Autodesk Fusion 360 part; units mm, degrees
note: some values were not read from the file. Chosen so that the rebuilt part matches the saved one: which bodies a step acts on.
(part 3 of 3)
  line L1048 (193.125, 122.3141) -> (193.125, 116.0647)
  line L1049 (193.125, 116.0647) -> (191.8255, 116.0647)
  line L1050 (191.8255, 116.0647) -> (191.8255, 120.6243)
  line L1051 (191.8255, 120.6243) -> (189.2661, 120.6243)
  line L1052 (189.2661, 120.6243) -> (189.2661, 116.8805)
  line L1053 (189.2661, 116.8805) -> (187.9666, 116.8805)
  line L1054 (187.9666, 116.8805) -> (187.9666, 120.6243)
  line L1055 (187.9666, 120.6243) -> (185.752, 120.6243)
  line L1056 (185.752, 120.6243) -> (185.752, 116.2104)
  line L1057 (185.752, 116.2104) -> (184.4524, 116.2104)
  line L1058 (184.4524, 116.2104) -> (184.4524, 122.3141)
  line L1059 (184.4524, 122.3141) -> (193.125, 122.3141)
  spline S282 degree 3 poles (193.2842, 101.9604) (193.2842, 99.8627) (192.1835, 98.6537) (189.8098, 98.6537) knots 0 0 0 0 1 1 1 1
  line L1060 (189.8098, 98.6537) -> (184.4525, 98.6537)
  line L1061 (184.4525, 98.6537) -> (184.4525, 100.2706)
  line L1062 (184.4525, 100.2706) -> (189.9292, 100.2706)
  spline S283 degree 3 poles (189.9292, 100.2706) (191.3481, 100.2706) (191.9448, 100.9261) (191.9448, 101.9604) knots 0 0 0 0 1 1 1 1
  spline S284 degree 3 poles (191.9448, 101.9604) (191.9448, 102.9801) (191.3481, 103.6065) (189.9292, 103.6065) knots 0 0 0 0 1 1 1 1
  line L1063 (189.9292, 103.6065) -> (184.4525, 103.6065)
  line L1064 (184.4525, 103.6065) -> (184.4525, 105.2963)
  line L1065 (184.4525, 105.2963) -> (189.8098, 105.2963)
  spline S285 degree 3 poles (189.8098, 105.2963) (192.1835, 105.2963) (193.2842, 104.0435) (193.2842, 101.9604) knots 0 0 0 0 1 1 1 1
  line L1066 (193.125, 87.7978) -> (193.125, 86.1809)
  line L1067 (193.125, 86.1809) -> (189.3324, 86.1809)
  spline S286 degree 3 poles (189.3324, 86.1809) (188.3644, 86.1809) (187.3301, 86.3411) (186.4018, 86.414) knots 0 0 0 0 1 1 1 1
  line L1068 (186.4018, 86.414) -> (186.4018, 86.3703)
  line L1069 (186.4018, 86.3703) -> (188.2451, 85.5108)
  line L1070 (188.2451, 85.5108) -> (193.125, 82.9906)
  line L1071 (193.125, 82.9906) -> (193.125, 81.2134)
  line L1072 (193.125, 81.2134) -> (184.4525, 81.2134)
  line L1073 (184.4525, 81.2134) -> (184.4525, 82.8304)
  line L1074 (184.4525, 82.8304) -> (188.2185, 82.8304)
  spline S287 degree 3 poles (188.2185, 82.8304) (189.1866, 82.8304) (190.2872, 82.6702) (191.1757, 82.5973) knots 0 0 0 0 1 1 1 1
  line L1075 (191.1757, 82.5973) -> (191.1757, 82.641)
  line L1076 (191.1757, 82.641) -> (189.3192, 83.5005)
  line L1077 (189.3192, 83.5005) -> (184.4525, 86.0207)
  line L1078 (184.4525, 86.0207) -> (184.4525, 87.7979)
  line L1079 (184.4525, 87.7979) -> (193.125, 87.7978)
  line L1080 (193.125, 70.212) -> (193.125, 68.493)
  line L1081 (193.125, 68.493) -> (190.5657, 68.493)
  line L1082 (190.5657, 68.493) -> (189.0009, 67.1383)
  line L1083 (189.0009, 67.1383) -> (193.125, 64.7347)
  line L1084 (193.125, 64.7347) -> (193.125, 62.8555)
  line L1085 (193.125, 62.8555) -> (187.8207, 66.104)
  line L1086 (187.8207, 66.104) -> (184.4525, 63.1614)
  line L1087 (184.4525, 63.1614) -> (184.4525, 65.0552)
  line L1088 (184.4525, 65.0552) -> (188.3909, 68.4494)
  line L1089 (188.3909, 68.4494) -> (188.3909, 68.4931)
  line L1090 (188.3909, 68.4931) -> (184.4525, 68.4931)
  line L1091 (184.4525, 68.4931) -> (184.4525, 70.212)
  line L1092 (184.4525, 70.212) -> (193.125, 70.212)
  spline S288 degree 3 poles (193.2842, 49.5524) (193.2842, 47.4547) (192.1835, 46.2456) (189.8098, 46.2456) knots 0 0 0 0 1 1 1 1
  line L1093 (189.8098, 46.2456) -> (184.4525, 46.2456)
  line L1094 (184.4525, 46.2456) -> (184.4525, 47.8626)
  line L1095 (184.4525, 47.8626) -> (189.9292, 47.8626)
  spline S289 degree 3 poles (189.9292, 47.8626) (191.3481, 47.8626) (191.9448, 48.5181) (191.9448, 49.5524) knots 0 0 0 0 1 1 1 1
  spline S290 degree 3 poles (191.9448, 49.5524) (191.9448, 50.5721) (191.3481, 51.1985) (189.9292, 51.1985) knots 0 0 0 0 1 1 1 1
  line L1096 (189.9292, 51.1985) -> (184.4525, 51.1985)
  line L1097 (184.4525, 51.1985) -> (184.4525, 52.8883)
  line L1098 (184.4525, 52.8883) -> (189.8098, 52.8883)
  spline S291 degree 3 poles (189.8098, 52.8883) (192.1835, 52.8883) (193.2842, 51.6355) (193.2842, 49.5524) knots 0 0 0 0 1 1 1 1
  line L1099 (193.125, 35.419) -> (193.125, 33.7292)
  line L1100 (193.125, 33.7292) -> (189.2794, 33.7292)
  line L1101 (189.2794, 33.7292) -> (189.2794, 30.4661)
  line L1102 (189.2794, 30.4661) -> (193.125, 30.4661)
  line L1103 (193.125, 30.4661) -> (193.125, 28.7763)
  line L1104 (193.125, 28.7763) -> (184.4525, 28.7763)
  line L1105 (184.4525, 28.7763) -> (184.4525, 30.4661)
  line L1106 (184.4525, 30.4661) -> (187.9401, 30.4661)
  line L1107 (187.9401, 30.4661) -> (187.9401, 33.7292)
  line L1108 (187.9401, 33.7292) -> (184.4525, 33.7292)
  line L1109 (184.4525, 33.7292) -> (184.4525, 35.419)
  line L1110 (184.4525, 35.419) -> (193.125, 35.419)
  line L1111 (193.125, 17.7748) -> (193.125, 16.085)
  line L1112 (193.125, 16.085) -> (189.7303, 16.085)
  line L1113 (189.7303, 16.085) -> (189.7303, 14.6574)
  line L1114 (189.7303, 14.6574) -> (193.125, 12.618)
  line L1115 (193.125, 12.618) -> (193.125, 10.7096)
  line L1116 (193.125, 10.7096) -> (189.5048, 12.9822)
  spline S292 degree 3 poles (189.5048, 12.9822) (189.1468, 11.8459) (188.3379, 11.0884) (187.0251, 11.0884) knots 0 0 0 0 1 1 1 1
  spline S293 degree 3 poles (187.0251, 11.0884) (185.089, 11.0884) (184.4525, 12.618) (184.4525, 14.5991) knots 0 0 0 0 1 1 1 1
  line L1117 (184.4525, 14.5991) -> (184.4525, 17.7748)
  line L1118 (184.4525, 17.7748) -> (193.125, 17.7748)
  line L1119 (188.5103, 16.085) -> (185.6857, 16.085)
  line L1120 (185.6857, 16.085) -> (185.6857, 14.7739)
  spline S294 degree 3 poles (185.6857, 14.7739) (185.6857, 13.4629) (186.0305, 12.7491) (187.0251, 12.7491) knots 0 0 0 0 1 1 1 1
  spline S295 degree 3 poles (187.0251, 12.7491) (188.0063, 12.7491) (188.5103, 13.4628) (188.5103, 14.7739) knots 0 0 0 0 1 1 1 1
  line L1121 (188.5103, 14.7739) -> (188.5103, 16.085)
  line L1122 (17.9457, 85.157) -> (17.9457, 83.9457)
  line L1123 (17.9457, 83.9457) -> (19.921, 83.9457)
  line L1124 (19.921, 83.9457) -> (19.921, 85.157)
  line L1125 (19.921, 85.157) -> (17.9457, 85.157)
  line L1126 (36.9623, 85.1886) -> (36.9623, 83.9773)
  line L1127 (36.9623, 83.9773) -> (38.9377, 83.9773)
  line L1128 (38.9377, 83.9773) -> (38.9377, 85.1886)
  line L1129 (38.9377, 85.1886) -> (36.9623, 85.1886)
  line L1130 (94.1637, 120.1259) -> (94.1637, 118.9147)
  line L1131 (94.1637, 118.9147) -> (96.1391, 118.9147)
  line L1132 (96.1391, 118.9147) -> (96.1391, 120.1259)
  line L1133 (96.1391, 120.1259) -> (94.1637, 120.1259)
  line L1134 (113.1344, 102.6647) -> (113.1344, 101.4534)
  line L1135 (113.1344, 101.4534) -> (115.1097, 101.4534)
  line L1136 (115.1097, 101.4534) -> (115.1097, 102.6647)
  line L1137 (115.1097, 102.6647) -> (113.1344, 102.6647)
  line L1138 (132.2327, 120.1342) -> (132.2327, 118.9229)
  line L1139 (132.2327, 118.9229) -> (134.208, 118.9229)
  line L1140 (134.208, 118.9229) -> (134.208, 120.1342)
  line L1141 (134.208, 120.1342) -> (132.2327, 120.1342)
  line L1142 (151.2434, 67.7051) -> (151.2434, 66.4938)
  line L1143 (151.2434, 66.4938) -> (153.2187, 66.4938)
  line L1144 (153.2187, 66.4938) -> (153.2187, 67.7051)
  line L1145 (153.2187, 67.7051) -> (151.2434, 67.7051)
  line L1146 (54.8062, 194.2009) -> (54.8062, 189.8962)
  line L1147 (54.8062, 189.8962) -> (56.5579, 189.8962)
  line L1148 (56.5579, 189.8962) -> (56.5579, 194.2009)
  line L1149 (56.5579, 194.2009) -> (54.8062, 194.2009)
  line L1150 (52.9054, 176.9634) -> (52.9054, 172.6586)
  line L1151 (52.9054, 172.6586) -> (54.6571, 172.6586)
  line L1152 (54.6571, 172.6586) -> (54.6571, 176.9634)
  line L1153 (54.6571, 176.9634) -> (52.9054, 176.9634)
  line L1154 (52.9657, 71.9243) -> (52.9657, 67.6195)
  line L1155 (52.9657, 67.6195) -> (54.7174, 67.6195)
  line L1156 (54.7174, 67.6195) -> (54.7174, 71.9243)
  line L1157 (54.7174, 71.9243) -> (52.9657, 71.9243)
  line L1158 (73.7065, 176.8402) -> (73.7065, 172.5355)
  line L1159 (73.7065, 172.5355) -> (75.4582, 172.5355)
  line L1160 (75.4582, 172.5355) -> (75.4582, 176.8402)
  line L1161 (75.4582, 176.8402) -> (73.7065, 176.8402)
  line L1162 (71.9934, 159.3938) -> (71.9934, 155.0891)
  line L1163 (71.9934, 155.0891) -> (73.7451, 155.0891)
  line L1164 (73.7451, 155.0891) -> (73.7451, 159.3938)
  line L1165 (73.7451, 159.3938) -> (71.9934, 159.3938)
  line L1166 (74.9914, 50.243) -> (74.9914, 49.0317)
  line L1167 (74.9914, 49.0317) -> (76.9667, 49.0317)
  line L1168 (76.9667, 49.0317) -> (76.9667, 50.243)
  line L1169 (76.9667, 50.243) -> (74.9914, 50.243)
  line L1170 (94.0892, 172.6027) -> (94.0892, 171.3914)
  line L1171 (94.0892, 171.3914) -> (96.0645, 171.3914)
  line L1172 (96.0645, 171.3914) -> (96.0645, 172.6027)
  line L1173 (96.0645, 172.6027) -> (94.0892, 172.6027)
  line L1174 (90.7444, 141.9078) -> (90.7444, 137.6031)
  line L1175 (90.7444, 137.6031) -> (92.4961, 137.6031)
  line L1176 (92.4961, 137.6031) -> (92.4961, 141.9078)
  line L1177 (92.4961, 141.9078) -> (90.7444, 141.9078)
  line L1178 (94.4867, 141.7101) -> (94.4867, 137.4054)
  line L1179 (94.4867, 137.4054) -> (96.2384, 137.4054)
  line L1180 (96.2384, 137.4054) -> (96.2384, 141.7101)
  line L1181 (96.2384, 141.7101) -> (94.4867, 141.7101)
  line L1182 (130.8687, 192.9954) -> (130.8687, 188.6906)
  line L1183 (130.8687, 188.6906) -> (132.6204, 188.6906)
  line L1184 (132.6204, 188.6906) -> (132.6204, 192.9954)
  line L1185 (132.6204, 192.9954) -> (130.8687, 192.9954)
  line L1186 (129.0766, 176.5504) -> (129.0766, 172.2456)
  line L1187 (129.0766, 172.2456) -> (130.8283, 172.2456)
  line L1188 (130.8283, 172.2456) -> (130.8283, 176.5504)
  line L1189 (130.8283, 176.5504) -> (129.0766, 176.5504)
  line L1190 (129.0502, 19.4531) -> (129.0502, 15.1484)
  line L1191 (129.0502, 15.1484) -> (130.8019, 15.1484)
  line L1192 (130.8019, 15.1484) -> (130.8019, 19.4531)
  line L1193 (130.8019, 19.4531) -> (129.0502, 19.4531)
  line L1194 (186.2217, 19.3094) -> (186.2217, 15.0047)
  line L1195 (186.2217, 15.0047) -> (187.9734, 15.0047)
  line L1196 (187.9734, 15.0047) -> (187.9734, 19.3094)
  line L1197 (187.9734, 19.3094) -> (186.2217, 19.3094)
  line L1198 (186.7062, 16.6912) -> (186.7062, 16.5235)
  line L1199 (186.7062, 16.5235) -> (186.8367, 16.5235)
  line L1200 (186.8367, 16.5235) -> (186.8367, 16.6912)
  line L1201 (186.8367, 16.6912) -> (186.7062, 16.6912)
  line L1202 (168.9096, 54.8468) -> (168.9096, 50.542)
  line L1203 (168.9096, 50.542) -> (170.6613, 50.542)
  line L1204 (170.6613, 50.542) -> (170.6613, 54.8468)
  line L1205 (170.6613, 54.8468) -> (168.9096, 54.8468)
  line L1206 (166.8948, 141.7101) -> (166.8948, 137.4054)
  line L1207 (166.8948, 137.4054) -> (168.6465, 137.4054)
  line L1208 (168.6465, 137.4054) -> (168.6465, 141.7101)
  line L1209 (168.6465, 141.7101) -> (166.8948, 141.7101)
  line L1210 (170.6898, 142.0396) -> (170.6898, 137.7348)
  line L1211 (170.6898, 137.7348) -> (172.4415, 137.7348)
  line L1212 (172.4415, 137.7348) -> (172.4415, 142.0396)
  line L1213 (172.4415, 142.0396) -> (170.6898, 142.0396)
sketch "Skizze5" plane through (0, 0, 0) normal (0, 0, 1) x (1, 0, 0)
  line L0 (18.65, 201.85, -10) -> (2.15, 185.35, -10)
  line L1 (2.15, 18.65, -10) -> (18.65, 2.15, -10)
  line L2 (2.15, 2.15) -> (2.15, 201.85)
  line L3 (18.65, 2.15) -> (2.15, 18.65)
  line L4 (2.15, 185.35) -> (18.65, 201.85)
  line L5 (2.15, 201.85) -> (201.85, 201.85)
  line L6 (201.85, 2.15) -> (2.15, 2.15)
  line L7 (24.7, 201.85) -> (24.7, 2.15)
  line L8 (25.7, 201.85) -> (25.7, 2.15)
  line L9 (43.9, 201.85) -> (43.9, 2.15)
  line L10 (44.9, 201.85) -> (44.9, 2.15)
  line L11 (63.1, 201.85) -> (63.1, 2.15)
  line L12 (64.1, 201.85) -> (64.1, 2.15)
  line L13 (82.3, 201.85) -> (82.3, 2.15)
  line L14 (83.3, 201.85) -> (83.3, 2.15)
  line L15 (101.5, 201.85) -> (101.5, 2.15)
  line L16 (102.5, 201.85) -> (102.5, 2.15)
  line L17 (120.7, 201.85) -> (120.7, 2.15)
  line L18 (121.7, 201.85) -> (121.7, 2.15)
  line L19 (159.1, 201.85) -> (159.1, 2.15)
  line L20 (160.1, 201.85) -> (160.1, 2.15)
  line L21 (178.3, 201.85) -> (178.3, 2.15)
  line L22 (179.3, 201.85) -> (179.3, 2.15)
  line L23 (139.9, 201.85) -> (139.9, 2.15)
  line L24 (140.9, 201.85) -> (140.9, 2.15)
  line L25 (201.85, 18.65) -> (185.35, 2.15)
  line L26 (201.85, 185.35) -> (185.35, 201.85)
  line L27 (198.5, 15.3) -> (198.5, 188.7)
  line L28 (197.5, 14.3) -> (197.5, 189.7)
  line L29 (201.85, 201.85) -> (201.85, 2.15)
  line L30 (6.5, 189.7) -> (6.5, 14.3)
  line L31 (5.5, 188.7) -> (5.5, 15.3)
  dimension "d39" = 1
  dimension "d40" = 1
  dimension "d41" = 1
  dimension "d42" = 1
  dimension "d43" = 1
  dimension "d44" = 1
  dimension "d45" = 1
  dimension "d46" = 1
  dimension "d49" = 18.2
  dimension "d50" = 18.2
  dimension "d53" = 18.2
  dimension "d54" = 18.2
  dimension "d55" = 18.2
  dimension "d58" = 1
  dimension "d60" = 18.2
  dimension "d61" = 18.2
  dimension "d63" = 18.2
  dimension "d65" = 1
  dimension "d66" = 18.2
  dimension "d67" = 2.7
  dimension "d96" = 1
  dimension "d97" = 18.2
  dimension "d98" = 3.35
  constraint coincident L5 L7.start
  constraint coincident L6 L7.end
  constraint perpendicular L6 L7
  constraint coincident L5 L8.start
  constraint coincident L6 L8.end
  constraint perpendicular L6 L8
  constraint coincident L5 L9.start
  constraint coincident L6 L9.end
  constraint perpendicular L6 L9
  constraint coincident L5 L10.start
  constraint coincident L6 L10.end
  constraint perpendicular L6 L10
  constraint coincident L5 L11.start
  constraint coincident L6 L11.end
  constraint perpendicular L6 L11
  constraint coincident L5 L12.start
  constraint coincident L6 L12.end
  constraint perpendicular L6 L12
  constraint coincident L5 L13.start
  constraint coincident L6 L13.end
  constraint perpendicular L6 L13
  constraint coincident L5 L14.start
  constraint coincident L6 L14.end
  constraint perpendicular L6 L14
  constraint coincident L5 L15.start
  constraint coincident L6 L15.end
  constraint perpendicular L6 L15
  constraint coincident L5 L16.start
  constraint coincident L6 L16.end
  constraint perpendicular L6 L16
  constraint coincident L5 L17.start
  constraint coincident L6 L17.end
  constraint perpendicular L6 L17
  constraint coincident L5 L18.start
  constraint coincident L6 L18.end
  constraint perpendicular L6 L18
  constraint coincident L5 L19.start
  constraint coincident L6 L19.end
  constraint perpendicular L6 L19
  constraint coincident L5 L20.start
  constraint coincident L6 L20.end
  constraint perpendicular L6 L20
  constraint coincident L5 L21.start
  constraint coincident L6 L21.end
  constraint perpendicular L6 L21
  constraint coincident L5 L22.start
  constraint coincident L6 L22.end
  constraint perpendicular L6 L22
  constraint coincident L5 L23.start
  constraint coincident L6 L23.end
  constraint perpendicular L6 L23
  constraint coincident L5 L24.start
  constraint coincident L6 L24.end
  constraint perpendicular L6 L24
  constraint coincident L25 L27.start
  constraint coincident L26 L27.end
  constraint vertical L27
  constraint coincident L25 L28.start
  constraint coincident L26 L28.end
  constraint parallel L27 L28
  constraint coincident L4 L30.start
  constraint coincident L3 L30.end
  constraint parallel L2 L30
  constraint coincident L4 L31.start
  constraint coincident L3 L31.end
  constraint parallel L30 L31
  measures "d39" distance of L7 L8
  measures "d40" distance of L9 L10
  measures "d41" distance of L11 L12
  measures "d42" distance of L13 L14
  measures "d43" distance of L15 L16
  measures "d44" distance of L17 L18
  measures "d45" distance of L19 L20
  measures "d46" distance of L21 L22
  measures "d49" distance of L10 L11
  measures "d50" distance of L12 L13
  measures "d53" distance of L8 L9
  measures "d54" distance of L14 L15
  measures "d55" distance of L16 L17
  measures "d58" distance of L23 L24
  measures "d60" distance of L18 L23
  measures "d61" distance of L19 L24
  measures "d63" distance of L20 L21
  measures "d65" distance of L27 L28
  measures "d66" distance of L22 L28
  measures "d96" distance of L30 L31
  measures "d97" distance of L7 L30
  measures "d98" distance of L2 L31
sketch "Skizze6" plane through (0, 0, 0) normal (0, 0, 1) x (1, 0, 0)
  line L0 (201.85, 18.65) -> (185.35, 2.15)
  line L1 (18.65, 2.15) -> (2.15, 18.65)
  line L2 (16.15, 4.65) -> (187.85, 4.65)
  line L3 (15.15, 5.65) -> (188.85, 5.65)
  line L4 (201.85, 2.15) -> (2.15, 2.15)
  line L5 (2.15, 185.35) -> (18.65, 201.85)
  line L6 (185.35, 201.85) -> (201.85, 185.35)
  line L7 (16.15, 199.35) -> (187.85, 199.35)
  line L8 (188.85, 198.35) -> (15.15, 198.35)
  line L9 (2.15, 201.85) -> (201.85, 201.85)
  line L10 (2.15, 2.15) -> (2.15, 201.85)
  line L11 (201.85, 201.85) -> (201.85, 2.15)
  line L12 (2.15, 23.75) -> (201.85, 23.75)
  line L13 (2.15, 40.25) -> (201.85, 40.25)
  line L14 (2.15, 41.25) -> (201.85, 41.25)
  line L15 (2.15, 57.75) -> (201.85, 57.75)
  line L16 (2.15, 58.75) -> (201.85, 58.75)
  line L17 (2.15, 75.25) -> (201.85, 75.25)
  line L18 (2.15, 76.25) -> (201.85, 76.25)
  line L19 (2.15, 92.75) -> (201.85, 92.75)
  line L20 (2.15, 93.75) -> (201.85, 93.75)
  line L21 (2.15, 111.25) -> (201.85, 111.25)
  line L22 (2.15, 110.25) -> (201.85, 110.25)
  line L23 (2.15, 127.75) -> (201.85, 127.75)
  line L24 (2.15, 128.75) -> (201.85, 128.75)
  line L25 (2.15, 145.25) -> (201.85, 145.25)
  line L26 (2.15, 146.25) -> (201.85, 146.25)
  line L27 (2.15, 162.75) -> (201.85, 162.75)
  line L28 (2.15, 163.75) -> (201.85, 163.75)
  line L29 (2.15, 181.25) -> (201.85, 181.25)
  line L30 (2.15, 180.25) -> (201.85, 180.25)
  line L31 (2.15, 22.75) -> (201.85, 22.75)
  line L32 (194.85, 181.25) -> (194.85, 22.75)
  line L33 (9.15, 181.3) -> (9.15, 22.7)
  dimension "d68" = 2.5
  dimension "d69" = 1
  dimension "d70" = 1
  dimension "d73" = 1
  dimension "d75" = 1
  dimension "d76" = 1
  dimension "d77" = 1
  dimension "d79" = 16.5
  dimension "d80" = 16.5
  dimension "d81" = 16.5
  dimension "d82" = 16.5
  dimension "d83" = 1
  dimension "d84" = 16.5
  dimension "d85" = 1
  dimension "d86" = 16.5
  dimension "d87" = 16.5
  dimension "d88" = 1
  dimension "d89" = 1
  dimension "d90" = 16.5
  dimension "d92" = 1
  dimension "d93" = 16.5
  dimension "d94" = 17.1
  dimension "d95" = 2.25
  dimension "d103" = 1
  dimension "d104" = 17.1
  dimension "d194" = 7
  dimension "d195" = 7
  constraint coincident L1 L2.start
  constraint coincident L0 L2.end
  constraint coincident L1 L3.start
  constraint coincident L0 L3.end
  constraint parallel L2 L3
  constraint coincident L5 L7.start
  constraint coincident L6 L7.end
  constraint coincident L6 L8.start
  constraint coincident L5 L8.end
  constraint parallel L7 L8
  constraint coincident L10 L12.start
  constraint coincident L11 L12.end
  constraint perpendicular L11 L12
  constraint coincident L10 L13.start
  constraint coincident L11 L13.end
  constraint perpendicular L11 L13
  constraint coincident L10 L14.start
  constraint perpendicular L10 L14
  constraint coincident L10 L15.start
  constraint perpendicular L10 L15
  constraint coincident L10 L16.start
  constraint coincident L11 L16.end
  constraint perpendicular L11 L16
  constraint coincident L10 L17.start
  constraint coincident L11 L17.end
  constraint perpendicular L11 L17
  constraint coincident L10 L18.start
  constraint coincident L11 L18.end
  constraint perpendicular L11 L18
  constraint coincident L10 L19.start
  constraint coincident L11 L19.end
  constraint perpendicular L11 L19
  constraint coincident L10 L20.start
  constraint coincident L11 L20.end
  constraint perpendicular L11 L20
  constraint coincident L10 L21.start
  constraint coincident L11 L21.end
  constraint perpendicular L11 L21
  constraint coincident L10 L22.start
  constraint coincident L11 L22.end
  constraint perpendicular L11 L22
  constraint coincident L10 L23.start
  constraint coincident L11 L23.end
  constraint perpendicular L11 L23
  constraint coincident L10 L24.start
  constraint coincident L11 L24.end
  constraint perpendicular L11 L24
  constraint coincident L10 L25.start
  constraint coincident L11 L25.end
  constraint perpendicular L11 L25
  constraint coincident L10 L26.start
  constraint coincident L11 L26.end
  constraint perpendicular L11 L26
  constraint coincident L10 L27.start
  constraint coincident L11 L27.end
  constraint perpendicular L11 L27
  constraint coincident L10 L28.start
  constraint perpendicular L10 L28
  constraint coincident L10 L29.start
  constraint coincident L11 L29.end
  constraint perpendicular L11 L29
  constraint coincident L10 L30.start
  constraint coincident L11 L30.end
  constraint perpendicular L11 L30
  constraint coincident L10 L31.start
  constraint coincident L11 L31.end
  constraint perpendicular L11 L31
  constraint coincident L29 L32.start
  constraint coincident L31 L32.end
  constraint perpendicular L31 L32
  measures "d68" distance of L2 L4
  measures "d69" distance of L2 L3
  measures "d70" distance of L7 L8
  measures "d73" distance of L13 L14
  measures "d75" distance of L15 L16
  measures "d76" distance of L17 L18
  measures "d77" distance of L19 L20
  measures "d79" distance of L12 L13
  measures "d80" distance of L14 L15
  measures "d81" distance of L16 L17
  measures "d82" distance of L18 L19
  measures "d83" distance of L21 L22
  measures "d84" distance of L20 L22
  measures "d85" distance of L23 L24
  measures "d86" distance of L21 L23
  measures "d87" distance of L24 L25
  measures "d88" distance of L25 L26
  measures "d89" distance of L27 L28
  measures "d90" distance of L26 L27
  measures "d92" distance of L29 L30
  measures "d93" distance of L28 L30
  measures "d94" distance of L8 L29
  measures "d103" distance of L12 L31
  measures "d104" distance of L3 L31
  measures "d194" distance of L11 L32
  measures "d195" distance of L10 L33
extrude "Extrusion3" add sketch "Skizze2" along normal blind 9 contours L0 L3 L4 L5 L6 L7 | L0 L1 L7 L12 L13 | L2 L3 L6 L8 L9 | L1 L2 L10 L11 bodies 1
extrude "Extrusion4" add sketch "Skizze5" against normal blind 9 contours L3 L4 L30 L31 | L5 L6 L7 L8 | L5 L6 L9 L10 | L5 L6 L11 L12 | L5 L6 L13 L14 | L5 L6 L15 L16 | L5 L6 L17 L18 | L5 L6 L23 L24 | L5 L6 L19 L20 | L5 L6 L21 L22 | L25 L26 L27 L28 bodies 1
extrude "Extrusion5" add sketch "Skizze6" against normal blind 9 separate body contours L0 L1 L2 L3 | L11 L12 L31 L32 | L12 L31 L32 L33 | L11 L13 L14 L32 | L10 L12 L31 L33 | L13 L14 L32 L33 | L11 L15 L16 L32 | L10 L13 L14 L33 | L15 L16 L32 L33 | L11 L17 L18 L32 | L10 L15 L16 L33 | L17 L18 L32 L33 | L11 L19 L20 L32 | L10 L17 L18 L33 | L19 L20 L32 L33 | L11 L21 L22 L32 | L10 L19 L20 L33 | L21 L22 L32 L33 | L11 L23 L24 L32 | L10 L21 L22 L33 | L23 L24 L32 L33 | L11 L25 L26 L32 | L10 L23 L24 L33 | L25 L26 L32 L33 | L11 L27 L28 L32 | L10 L25 L26 L33 | L27 L28 L32 L33 | L11 L29 L30 L32 | L10 L27 L28 L33 | L29 L30 L32 L33 | L10 L29 L30 L33 | L5 L6 L7 L8 makes body 2 at (68.7167, 40.25, -3) makes body 3 at (68.7167, 110.25, -3) makes body 4 at (68.7167, 180.25, -3) makes body 5 at (68.7167, 162.75, -3) makes body 6 at (68.7167, 92.75, -3) makes body 7 at (68.7167, 22.75, -3) makes body 8 at (68.7167, 57.75, -3) makes body 9 at (68.7167, 127.75, -3) makes body 10 at (130.95, 198.35, -3) makes body 11 at (68.7167, 145.25, -3) makes body 12 at (68.7167, 75.25, -3) makes body 13 at (73.05, 5.65, -6)
sketch "Skizze7" plane through (0, 0, 4) normal (0, 0, 1) x (-1, 0, 0)
  line L0 (-2.15, -2.15) -> (-201.85, -2.15)
  line L1 (-201.85, -2.15) -> (-201.85, -201.85)
  line L2 (-201.85, -201.85) -> (-2.15, -201.85)
  line L3 (-2.15, -201.85) -> (-2.15, -2.15)
  circle A0 centre (-7.65, -7.65) radius 5.5
  line L4 (-3.7553, -7.6507) -> (-7.6477, -11.5365)
  line L5 (-7.6477, -11.5365) -> (-11.5417, -7.6523)
  line L6 (-11.5417, -7.6523) -> (-7.6034, -3.7147)
  line L7 (-7.6034, -3.7147) -> (-3.7553, -7.6507)
  circle A1 centre (-196.35, -7.65) radius 5.5
  line L8 (-196.4069, -11.5386) -> (-200.2387, -7.5931)
  line L9 (-192.4558, -7.7125) -> (-196.4069, -11.5386)
  line L10 (-196.2466, -3.7162) -> (-192.4558, -7.7125)
  line L11 (-200.2387, -7.5931) -> (-196.2466, -3.7162)
  line L12 (-7.7086, -192.4266) -> (-3.7586, -196.2464)
  line L13 (-3.7586, -196.2464) -> (-7.5504, -200.2304)
  line L14 (-11.5453, -196.45) -> (-7.7086, -192.4266)
  line L15 (-7.5504, -200.2304) -> (-11.5453, -196.45)
  circle A2 centre (-7.65, -196.35) radius 5.5
  line L16 (-195.8812, -192.0876) -> (-192.4548, -196.4254)
  line L17 (-192.4548, -196.4254) -> (-196.4237, -200.233)
  line L18 (-200.2438, -196.2761) -> (-195.8812, -192.0876)
  line L19 (-196.4237, -200.233) -> (-200.2438, -196.2761)
  circle A3 centre (-196.35, -196.35) radius 5.5
  dimension "d107" = 11
  dimension "d109" = 5.5
  dimension "d112" = 5.5
  dimension "d113" = 5.5
  dimension "d115" = 5.5
  dimension "d117" = 2.75
  dimension "d118" = 2.75
  dimension "d121" = 11
  dimension "d122" = 5.5
  dimension "d123" = 5.5
  dimension "d124" = 2.75
  dimension "d125" = 2.75
  dimension "d126" = 5.5
  dimension "d127" = 5.5
  dimension "d128" = 11
  dimension "d129" = 5.5
  dimension "d130" = 5.5
  dimension "d131" = 2.75
  dimension "d132" = 2.75
  dimension "d133" = 11
  dimension "d134" = 5.5
  dimension "d135" = 5.5
  dimension "d136" = 2.75
  dimension "d137" = 2.75
  dimension "d138" = 5.5
  dimension "d139" = 5.5
  dimension "d140" = 5.5
  dimension "d141" = 5.5
  measures "d107" diameter of A0
  measures "d109" distance of L0 A0.centre
  measures "d112" distance of L4.start L4.end
  measures "d113" distance of L4.end L5.end
  measures "d115" distance of L3 A0.centre
  measures "d117" distance of A0.centre L5
  measures "d118" distance of A0.centre L6
  measures "d121" diameter of A1
  measures "d122" distance of L9.start L8.start
  measures "d123" distance of L8.end L8.start
  measures "d124" distance of A1.centre L8
  measures "d125" distance of A1.centre L11
  measures "d126" distance of L0 A1.centre
  measures "d127" distance of L1 A1.centre
  measures "d128" diameter of A2
  measures "d129" distance of L12.end L13.end
  measures "d130" distance of L14.start L13.end
  measures "d131" distance of A2.centre L15
  measures "d132" distance of A2.centre L14
  measures "d133" diameter of A3
  measures "d134" distance of L16.end L17.end
  measures "d135" distance of L18.start L17.end
  measures "d136" distance of A3.centre L19
  measures "d137" distance of A3.centre L18
  measures "d138" distance of L1 A3.centre
  measures "d139" distance of L2 A3.centre
  measures "d140" distance of L3 A2.centre
  measures "d141" distance of L2 A2.centre
extrude "Extrusion9" cut sketch "Skizze7" against normal blind 2 contours A0 | A1 | A2 | A3 bodies 1
extrude "Extrusion10" cut sketch "Skizze7" against normal blind 5 contours L4 L5 L6 L7 | L8 L9 L10 L11 | L12 L13 L14 L15 | L16 L17 L18 L19 bodies 1
sketch "Skizze8" plane through (0, 0, 4) normal (0, 0, 1) x (-1, 0, 0)
  arc A0 (-196.35, -201.85) -> (-201.85, -196.35) centre (-196.35, -196.35) ccw
  line L0 (-196.35, -201.85) -> (-7.65, -201.85)
  arc A1 (-2.15, -196.35) -> (-7.65, -201.85) centre (-7.65, -196.35) ccw
  line L1 (-2.15, -196.35) -> (-2.15, -7.65)
  arc A2 (-7.65, -2.15) -> (-2.15, -7.65) centre (-7.65, -7.65) ccw
  line L2 (-7.65, -2.15) -> (-196.35, -2.15)
  arc A3 (-201.85, -7.65) -> (-196.35, -2.15) centre (-196.35, -7.65) ccw
  line L3 (-201.85, -7.65) -> (-201.85, -196.35)
  line L4 (-22, -2.15) -> (-22, -201.85)
  line L5 (-11, -2.15) -> (-11, -201.85)
  line L6 (-2.15, -2.15) -> (-2.15, -201.85)
  line L7 (-41, -2.15) -> (-41, -201.85)
  line L8 (-30, -2.15) -> (-30, -201.85)
  line L9 (-60, -2.15) -> (-60, -201.85)
  line L10 (-49, -2.15) -> (-49, -201.85)
  line L11 (-79, -2.15) -> (-79, -201.85)
  line L12 (-68, -2.15) -> (-68, -201.85)
  line L13 (-98, -2.15) -> (-98, -201.85)
  line L14 (-87, -2.15) -> (-87, -201.85)
  line L15 (-117, -2.15) -> (-117, -201.85)
  line L16 (-106, -2.15) -> (-106, -201.85)
  line L17 (-136, -2.15) -> (-136, -201.85)
  line L18 (-125, -2.15) -> (-125, -201.85)
  line L19 (-155, -2.15) -> (-155, -201.85)
  line L20 (-144, -2.15) -> (-144, -201.85)
  line L21 (-174, -2.15) -> (-174, -201.85)
  line L22 (-163, -2.15) -> (-163, -201.85)
  line L23 (-193, -2.15) -> (-193, -201.85)
  line L24 (-182, -2.15) -> (-182, -201.85)
  line L25 (-201.85, -201.85) -> (-201.85, -2.15)
  line L26 (-4.15, -2.15) -> (-4.15, -201.85)
  line L27 (-9.15, -2.15) -> (-9.15, -201.85)
  line L28 (-4.15, -199.85) -> (-199.85, -199.85)
  line L29 (-4.15, -194.85) -> (-199.85, -194.85)
  line L30 (-4.15, -4.15) -> (-199.85, -4.15)
  line L31 (-4.15, -9.15) -> (-199.85, -9.15)
  line L32 (-199.85, -2.15) -> (-199.85, -201.85)
  line L33 (-194.85, -2.15) -> (-194.85, -201.85)
  dimension "d148" = 11
  dimension "d149" = 8.85
  dimension "d151" = 11
  dimension "d152" = 11
  dimension "d153" = 11
  dimension "d154" = 11
  dimension "d155" = 11
  dimension "d156" = 11
  dimension "d157" = 11
  dimension "d158" = 11
  dimension "d159" = 11
  dimension "d160" = 8.85
  dimension "d161" = 8
  dimension "d162" = 8
  dimension "d163" = 8
  dimension "d164" = 8
  dimension "d165" = 8
  dimension "d166" = 8
  dimension "d167" = 8
  dimension "d168" = 8
  dimension "d169" = 7
  dimension "d178" = 2
  dimension "d179" = 5
  dimension "d182" = 2
  dimension "d183" = 5
  dimension "d184" = 5
  dimension "d185" = 2
  dimension "d186" = 2
  dimension "d187" = 5
  constraint coincident L2 L4.start
  constraint coincident L0 L4.end
  constraint perpendicular L0 L4
  constraint coincident L26 L28.start
  measures "d148" distance of L4 L5
  measures "d149" distance of L5 L6
  measures "d151" distance of L7 L8
  measures "d152" distance of L9 L10
  measures "d153" distance of L11 L12
  measures "d154" distance of L13 L14
  measures "d155" distance of L15 L16
  measures "d156" distance of L17 L18
  measures "d157" distance of L19 L20
  measures "d158" distance of L21 L22
  measures "d159" distance of L23 L24
  measures "d160" distance of L23 L25
  measures "d161" distance of L4 L8
  measures "d162" distance of L7 L10
  measures "d163" distance of L9 L12
  measures "d164" distance of L11 L14
  measures "d165" distance of L13 L16
  measures "d166" distance of L15 L18
  measures "d167" distance of L17 L20
  measures "d168" distance of L19 L22
  measures "d178" distance of L6 L26
  measures "d179" distance of L26 L27
  measures "d182" distance of L0 L28
  measures "d183" distance of L28 L29
  measures "d184" distance of L30 L31
  measures "d185" distance of L2 L30
  measures "d186" distance of L25 L32
  measures "d187" distance of L32 L33
extrude "Extrusion11" cut sketch "Skizze8" against normal blind 2 contours L23 L28 L29 L33 | L28 L29 L32 L33 | A0 L23 L28 L29 | A0 L24 L28 L29 | A0 L29 L32 L33 | A0 L23 L29 | A0 A3 L23 L24 L29 L31 | L21 L24 L28 L29 | A0 A3 L32 L33 | L21 L22 L28 L29 | A3 L31 L32 L33 | A3 L23 L31 | A3 L24 L30 L31 | L21 L24 L30 L31 | L21 L22 L29 L31 | L19 L22 L28 L29 | L23 L30 L31 L33 | L30 L31 L32 L33 | A3 L23 L30 L31 | L21 L22 L30 L31 | L19 L20 L28 L29 | L19 L22 L30 L31 | L19 L20 L29 L31 | L17 L20 L28 L29 | L19 L20 L30 L31 | L17 L18 L28 L29 | L17 L20 L30 L31 | L17 L18 L29 L31 | L15 L18 L28 L29 | L17 L18 L30 L31 | L15 L16 L28 L29 | L15 L18 L30 L31 | L15 L16 L29 L31 | L13 L16 L28 L29 | L15 L16 L30 L31 | L13 L14 L28 L29 | L13 L16 L30 L31 | L13 L14 L29 L31 | L11 L14 L28 L29 | L13 L14 L30 L31 | L11 L12 L28 L29 | L11 L14 L30 L31 | L11 L12 L29 L31 | L9 L12 L28 L29 | L11 L12 L30 L31 | L9 L10 L28 L29 | L9 L12 L30 L31 | L9 L10 L29 L31 | L7 L10 L28 L29 | L9 L10 L30 L31 | L7 L8 L28 L29 | L7 L10 L30 L31 | L7 L8 L29 L31 | L4 L8 L28 L29 | L7 L8 L30 L31 | A1 L4 L28 L29 | L4 L8 L30 L31 | A1 A2 L4 L5 L29 L31 | A1 L5 L28 L29 | A2 L4 L30 L31 | A1 L5 L29 | L5 L27 L28 L29 | A2 L5 L31 | A2 L5 L30 L31 | L26 L27 L28 L29 | L5 L27 L30 L31 | A1 A2 L26 L27 | A1 L26 L27 L29 | A2 L26 L27 L31 | L26 L27 L30 L31 bodies 1
sketch "Skizze10" plane through (0, 0, 4) normal (0, 0, 1) x (-1, 0, 0)
  circle A0 centre (-16.5, -18.5) radius 4
  line L0 (-11, -2.15) -> (-11, -201.85)
  line L1 (-7.65, -2.15) -> (-196.35, -2.15)
  circle A1 centre (-16.5, -18.5) radius 4
  circle A2 centre (-16.5, -35.2) radius 4
  circle A3 centre (-16.5, -51.9) radius 4
  circle A4 centre (-16.5, -68.6) radius 4
  circle A5 centre (-16.5, -85.3) radius 4
  circle A6 centre (-16.5, -102) radius 4
  circle A7 centre (-16.5, -118.7) radius 4
  circle A8 centre (-16.5, -135.4) radius 4
  circle A9 centre (-16.5, -135.4) radius 4
  circle A10 centre (-16.5, -152.1) radius 4
  circle A11 centre (-16.5, -168.8) radius 4
  circle A12 centre (-16.5, -185.5) radius 4
  circle A13 centre (-35.5, -18.5) radius 4
  circle A14 centre (-35.5, -35.2) radius 4
  circle A15 centre (-35.5, -51.9) radius 4
  circle A16 centre (-35.5, -68.6) radius 4
  circle A17 centre (-35.5, -85.3) radius 4
  circle A18 centre (-35.5, -102) radius 4
  circle A19 centre (-35.5, -118.7) radius 4
  circle A20 centre (-35.5, -135.4) radius 4
  circle A21 centre (-35.5, -152.1) radius 4
  circle A22 centre (-35.5, -168.8) radius 4
  circle A23 centre (-35.5, -185.5) radius 4
  circle A24 centre (-54.5, -18.5) radius 4
  circle A25 centre (-54.5, -35.2) radius 4
  circle A26 centre (-54.5, -51.9) radius 4
  circle A27 centre (-54.5, -68.6) radius 4
  circle A28 centre (-54.5, -85.3) radius 4
  circle A29 centre (-54.5, -102) radius 4
  circle A30 centre (-54.5, -118.7) radius 4
  circle A31 centre (-54.5, -135.4) radius 4
  circle A32 centre (-54.5, -152.1) radius 4
  circle A33 centre (-54.5, -168.8) radius 4
  circle A34 centre (-54.5, -185.5) radius 4
  circle A35 centre (-73.5, -18.5) radius 4
  circle A36 centre (-73.5, -35.2) radius 4
  circle A37 centre (-73.5, -51.9) radius 4
  circle A38 centre (-73.5, -68.6) radius 4
  circle A39 centre (-73.5, -85.3) radius 4
  circle A40 centre (-73.5, -102) radius 4
  circle A41 centre (-73.5, -118.7) radius 4
  circle A42 centre (-73.5, -135.4) radius 4
  circle A43 centre (-73.5, -152.1) radius 4
  circle A44 centre (-73.5, -168.8) radius 4
  circle A45 centre (-73.5, -185.5) radius 4
  circle A46 centre (-92.5, -18.5) radius 4
  circle A47 centre (-92.5, -35.2) radius 4
  circle A48 centre (-92.5, -51.9) radius 4
  circle A49 centre (-92.5, -68.6) radius 4
  circle A50 centre (-92.5, -85.3) radius 4
  circle A51 centre (-92.5, -102) radius 4
  circle A52 centre (-92.5, -118.7) radius 4
  circle A53 centre (-92.5, -135.4) radius 4
  circle A54 centre (-92.5, -152.1) radius 4
  circle A55 centre (-92.5, -168.8) radius 4
  circle A56 centre (-92.5, -185.5) radius 4
  circle A57 centre (-111.5, -18.5) radius 4
  circle A58 centre (-111.5, -35.2) radius 4
  circle A59 centre (-111.5, -51.9) radius 4
  circle A60 centre (-111.5, -68.6) radius 4
  circle A61 centre (-111.5, -85.3) radius 4
  circle A62 centre (-111.5, -102) radius 4
  circle A63 centre (-111.5, -118.7) radius 4
  circle A64 centre (-111.5, -135.4) radius 4
  circle A65 centre (-111.5, -152.1) radius 4
  circle A66 centre (-111.5, -168.8) radius 4
  circle A67 centre (-111.5, -185.5) radius 4
  circle A68 centre (-130.5, -18.5) radius 4
  circle A69 centre (-130.5, -35.2) radius 4
  circle A70 centre (-130.5, -51.9) radius 4
  circle A71 centre (-130.5, -68.6) radius 4
  circle A72 centre (-130.5, -85.3) radius 4
  circle A73 centre (-130.5, -102) radius 4
  circle A74 centre (-130.5, -118.7) radius 4
  circle A75 centre (-130.5, -135.4) radius 4
  circle A76 centre (-130.5, -152.1) radius 4
  circle A77 centre (-130.5, -168.8) radius 4
  circle A78 centre (-130.5, -185.5) radius 4
  circle A79 centre (-149.5, -18.5) radius 4
  circle A80 centre (-149.5, -35.2) radius 4
  circle A81 centre (-149.5, -51.9) radius 4
  circle A82 centre (-149.5, -68.6) radius 4
  circle A83 centre (-149.5, -85.3) radius 4
  circle A84 centre (-149.5, -102) radius 4
  circle A85 centre (-149.5, -118.7) radius 4
  circle A86 centre (-149.5, -135.4) radius 4
  circle A87 centre (-149.5, -152.1) radius 4
  circle A88 centre (-149.5, -168.8) radius 4
  circle A89 centre (-149.5, -185.5) radius 4
  circle A90 centre (-168.5, -18.5) radius 4
  circle A91 centre (-168.5, -35.2) radius 4
  circle A92 centre (-168.5, -51.9) radius 4
  circle A93 centre (-168.5, -68.6) radius 4
  circle A94 centre (-168.5, -85.3) radius 4
  circle A95 centre (-168.5, -102) radius 4
  circle A96 centre (-168.5, -118.7) radius 4
  circle A97 centre (-168.5, -135.4) radius 4
  circle A98 centre (-168.5, -152.1) radius 4
  circle A99 centre (-168.5, -168.8) radius 4
  circle A100 centre (-168.5, -185.5) radius 4
  circle A101 centre (-187.5, -18.5) radius 4
  circle A102 centre (-187.5, -35.2) radius 4
  circle A103 centre (-187.5, -51.9) radius 4
  circle A104 centre (-187.5, -68.6) radius 4
  circle A105 centre (-187.5, -85.3) radius 4
  circle A106 centre (-187.5, -102) radius 4
  circle A107 centre (-187.5, -118.7) radius 4
  circle A108 centre (-187.5, -135.4) radius 4
  circle A109 centre (-187.5, -152.1) radius 4
  circle A110 centre (-187.5, -168.8) radius 4
  circle A111 centre (-187.5, -185.5) radius 4
  dimension "d222" = 8
  dimension "d223" = 5.5
  dimension "d224" = 16.35
  dimension "d226" = 8
  dimension "d227" = 8
  dimension "d228" = 8
  dimension "d229" = 8
  dimension "d230" = 8
  dimension "d231" = 8
  dimension "d232" = 8
  dimension "d233" = 8
  dimension "d234" = 8
  dimension "d235" = 8
  dimension "d236" = 8
  dimension "d237" = 8
  dimension "d238" = 8
  dimension "d239" = 8
  dimension "d240" = 8
  dimension "d241" = 8
  dimension "d242" = 8
  dimension "d243" = 8
  dimension "d244" = 8
  dimension "d245" = 8
  dimension "d246" = 8
  dimension "d247" = 8
  dimension "d248" = 8
  dimension "d249" = 8
  dimension "d250" = 8
  dimension "d251" = 8
  dimension "d252" = 8
  dimension "d253" = 8
  dimension "d254" = 8
  dimension "d255" = 8
  dimension "d256" = 8
  dimension "d257" = 8
  dimension "d258" = 8
  dimension "d259" = 8
  dimension "d260" = 8
  dimension "d261" = 8
  dimension "d262" = 8
  dimension "d263" = 8
  dimension "d264" = 8
  dimension "d265" = 8
  dimension "d266" = 8
  dimension "d267" = 8
  dimension "d268" = 8
  dimension "d269" = 8
  dimension "d270" = 8
  dimension "d271" = 8
  dimension "d272" = 8
  dimension "d273" = 8
  dimension "d274" = 8
  dimension "d275" = 8
  dimension "d276" = 8
  dimension "d277" = 8
  dimension "d278" = 8
  dimension "d279" = 8
  dimension "d280" = 8
  dimension "d281" = 8
  dimension "d282" = 8
  dimension "d283" = 8
  dimension "d284" = 8
  dimension "d285" = 8
  dimension "d286" = 8
  dimension "d287" = 8
  dimension "d288" = 8
  dimension "d289" = 8
  dimension "d290" = 8
  dimension "d291" = 8
  dimension "d292" = 8
  dimension "d293" = 8
  dimension "d294" = 8
  dimension "d295" = 8
  dimension "d296" = 8
  dimension "d297" = 8
  dimension "d298" = 8
  dimension "d299" = 8
  dimension "d300" = 8
  dimension "d301" = 8
  dimension "d302" = 8
  dimension "d303" = 8
  dimension "d304" = 8
  dimension "d305" = 8
  dimension "d306" = 8
  dimension "d307" = 8
  dimension "d308" = 8
  dimension "d309" = 8
  dimension "d310" = 8
  dimension "d311" = 8
  dimension "d312" = 8
  dimension "d313" = 8
  dimension "d314" = 8
  dimension "d315" = 8
  dimension "d316" = 8
  dimension "d317" = 8
  dimension "d318" = 8
  dimension "d319" = 8
  dimension "d320" = 8
  dimension "d321" = 8
  dimension "d322" = 8
  dimension "d323" = 8
  dimension "d324" = 8
  dimension "d325" = 8
  dimension "d326" = 8
  dimension "d327" = 8
  dimension "d328" = 8
  dimension "d329" = 8
  dimension "d330" = 8
  dimension "d331" = 8
  dimension "d332" = 8
  dimension "d333" = 8
  dimension "d334" = 8
  dimension "d335" = 8
  dimension "d336" = 8
  measures "d222" diameter of A0
  measures "d223" distance of A0.centre L0
  measures "d224" distance of A0.centre L1
  measures "d226" diameter of A1
  measures "d227" diameter of A2
  measures "d228" diameter of A3
  measures "d229" diameter of A4
  measures "d230" diameter of A5
  measures "d231" diameter of A6
  measures "d232" diameter of A7
  measures "d233" diameter of A8
  measures "d234" diameter of A9
  measures "d235" diameter of A10
  measures "d236" diameter of A11
  measures "d237" diameter of A12
  measures "d238" diameter of A13
  measures "d239" diameter of A14
  measures "d240" diameter of A15
  measures "d241" diameter of A16
  measures "d242" diameter of A17
  measures "d243" diameter of A18
  measures "d244" diameter of A19
  measures "d245" diameter of A20
  measures "d246" diameter of A21
  measures "d247" diameter of A22
  measures "d248" diameter of A23
  measures "d249" diameter of A24
  measures "d250" diameter of A25
  measures "d251" diameter of A26
  measures "d252" diameter of A27
  measures "d253" diameter of A28
  measures "d254" diameter of A29
  measures "d255" diameter of A30
  measures "d256" diameter of A31
  measures "d257" diameter of A32
  measures "d258" diameter of A33
  measures "d259" diameter of A34
  measures "d260" diameter of A35
  measures "d261" diameter of A36
  measures "d262" diameter of A37
  measures "d263" diameter of A38
  measures "d264" diameter of A39
  measures "d265" diameter of A40
  measures "d266" diameter of A41
  measures "d267" diameter of A42
  measures "d268" diameter of A43
  measures "d269" diameter of A44
  measures "d270" diameter of A45
  measures "d271" diameter of A46
  measures "d272" diameter of A47
  measures "d273" diameter of A48
  measures "d274" diameter of A49
  measures "d275" diameter of A50
  measures "d276" diameter of A51
  measures "d277" diameter of A52
  measures "d278" diameter of A53
  measures "d279" diameter of A54
  measures "d280" diameter of A55
  measures "d281" diameter of A56
  measures "d282" diameter of A57
  measures "d283" diameter of A58
  measures "d284" diameter of A59
  measures "d285" diameter of A60
  measures "d286" diameter of A61
  measures "d287" diameter of A62
  measures "d288" diameter of A63
  measures "d289" diameter of A64
  measures "d290" diameter of A65
  measures "d291" diameter of A66
  measures "d292" diameter of A67
  measures "d293" diameter of A68
  measures "d294" diameter of A69
  measures "d295" diameter of A70
  measures "d296" diameter of A71
  measures "d297" diameter of A72
  measures "d298" diameter of A73
  measures "d299" diameter of A74
  measures "d300" diameter of A75
  measures "d301" diameter of A76
  measures "d302" diameter of A77
  measures "d303" diameter of A78
  measures "d304" diameter of A79
  measures "d305" diameter of A80
  measures "d306" diameter of A81
  measures "d307" diameter of A82
  measures "d308" diameter of A83
  measures "d309" diameter of A84
  measures "d310" diameter of A85
  measures "d311" diameter of A86
  measures "d312" diameter of A87
  measures "d313" diameter of A88
  measures "d314" diameter of A89
  measures "d315" diameter of A90
  measures "d316" diameter of A91
  measures "d317" diameter of A92
  measures "d318" diameter of A93
  measures "d319" diameter of A94
  measures "d320" diameter of A95
  measures "d321" diameter of A96
  measures "d322" diameter of A97
  measures "d323" diameter of A98
  measures "d324" diameter of A99
  measures "d325" diameter of A100
  measures "d326" diameter of A101
  measures "d327" diameter of A102
  measures "d328" diameter of A103
  measures "d329" diameter of A104
  measures "d330" diameter of A105
  measures "d331" diameter of A106
  measures "d332" diameter of A107
  measures "d333" diameter of A108
  measures "d334" diameter of A109
  measures "d335" diameter of A110
  measures "d336" diameter of A111
extrude "Extrusion15" cut sketch "Skizze10" against normal blind 5 bodies 1
sketch "Skizze14" plane through (0, 0, 4) normal (0, 0, 1) x (-1, 0, 0)
  line L0 (-174, -9.15) -> (-182, -9.15)
  line L1 (-182, -9.15) -> (-182, -194.85)
  line L2 (-182, -194.85) -> (-174, -194.85)
  line L3 (-174, -194.85) -> (-174, -9.15)
  circle A0 centre (-121, -127) radius 3
  circle A1 centre (-121, -127) radius 1.5
  circle A2 centre (-82.6794, -83.4623) radius 3
  circle A3 centre (-82.6794, -83.4623) radius 1.5
  dimension "d361" = 6
  dimension "d362" = 3
  dimension "d363" = 6
  dimension "d364" = 3
  dimension "d365" = 58
  constraint concentric A2 A3
  measures "d361" diameter of A0
  measures "d362" diameter of A1
  measures "d363" diameter of A2
  measures "d364" diameter of A3
  measures "d365" distance of A0.centre A2.centre
extrude "Extrusion27" cut sketch "Skizze1" along normal blind 4 contours L3 L7 L16 L18 L19 | L6 L9 L10 L11 | L7 L16 L17 L18 | L5 L20 L21 L22 | L4 L13 L14 L15 bodies 1
extrude "Extrusion28" cut sketch "Skizze1" against normal blind 9 contours L6 L9 L10 L11 | L7 L16 L17 L18 | L5 L20 L21 L22 | L4 L13 L14 L15 bodies 1 10 13 makes body 15 at (41.35, 5.65, -3) makes body 14 at (159.3167, 198.35, -6)
fillet "Abrundung2" radius 4 36 edges at (98, 194.85, 3) (106, 194.85, 3) (117, 194.85, 3) (125, 194.85, 3) (87, 194.85, 3) (79, 194.85, 3) (68, 194.85, 3) (60, 194.85, 3) (49, 194.85, 3) (41, 194.85, 3) (30, 194.85, 3) (22, 194.85, 3) (136, 194.85, 3) (144, 194.85, 3) (155, 194.85, 3) (163, 194.85, 3) (174, 194.85, 3) (182, 194.85, 3) (182, 9.15, 3) (174, 9.15, 3) (163, 9.15, 3) (155, 9.15, 3) (144, 9.15, 3) (136, 9.15, 3) (125, 9.15, 3) (117, 9.15, 3) (106, 9.15, 3) (98, 9.15, 3) (87, 9.15, 3) (79, 9.15, 3) (60, 9.15, 3) (68, 9.15, 3) (49, 9.15, 3) (41, 9.15, 3) (30, 9.15, 3) (22, 9.15, 3) on bodies 1
fillet "Abrundung3" radius 0.9 8 edges at (194.85, 12.9415, 3) (193, 12.0121, 3) (194.85, 191.0585, 3) (193, 191.9879, 3) (11, 191.9879, 3) (9.15, 191.0585, 3) (11, 12.0121, 3) (9.15, 12.9415, 3) on bodies 1
fillet "Abrundung4" radius 2 8 edges at (8.5, 98.75, 1) (8.5, 105.25, 1) (93.75, 8.5, 1) (100.25, 8.5, 1) (93.75, 195.5, 1) (100.25, 195.5, 1) (195.5, 98.75, 1) (195.5, 105.25, 1) on bodies 1
sketch "Time Module Halterung" plane through (0, 0, 4) normal (0, 0, 1) x (-1, 0, 0)
  arc A0 (-136, -13.15) -> (-144, -13.15) centre (-140, -13.15) ccw
  line L0 (-144, -13.15) -> (-144, -190.85)
  arc A1 (-144, -190.85) -> (-136, -190.85) centre (-140, -190.85) ccw
  line L1 (-136, -190.85) -> (-136, -13.15)
  line L2 (-136, -77.499) -> (-144, -77.499)
  line L3 (-144, -77.499) -> (-144, -91.499)
  line L4 (-144, -91.499) -> (-136, -91.499)
  line L5 (-136, -91.499) -> (-136, -77.499)
  line L6 (-194.85, -76.25, -1) -> (-9.15, -76.25, -1)
  dimension "d406" = 14
  constraint horizontal L2
  constraint vertical L3
  constraint horizontal L4
  constraint vertical L5
  constraint coincident L0 L3.end
  constraint coincident L1 L2.start
  measures "d406" distance of L2 L4
extrude "Extrusion29" cut sketch "Time Module Halterung" against normal blind 3 contours L0 L1 L2 L3 L4 L5 bodies 1
extrude "Extrusion30" cut sketch "Skizze14" against normal blind 3 contours A1 | A3 bodies 1
fillet "Abrundung5" radius 0.5 4 edges at (201.85, 2.15, 2) (2.15, 2.15, 2) (2.15, 201.85, 2) (201.85, 201.85, 2) on bodies 1
